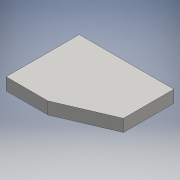
# Autodesk Inventor part: filter top
Saved by Autodesk Inventor 2016 SP1 (Build 200210100, 210)
## iProperties
Created: 2016-05-25
Part Number: filter top
Material: Generic
Document SubType Name: Modeling
Designer: ubik
Density: 1 g/cm^3
Appearance: Default
Author: ubik
Autodesk Inventor part; units mm, degrees
ref_plane "YZ Plane" through (0, 0, 0) normal (1, 0, 0) x (0, 1, 0)
ref_plane "XZ Plane" through (0, 0, 0) normal (0, 1, 0) x (-1, 0, 0)
ref_plane "XY Plane" through (0, 0, 0) normal (0, 0, 1) x (1, 0, 0)
sketch "Sketch1" plane through (0, 0, 0) normal (0, 0, 1) x (1, 0, 0)
  line L0 (-136, 105) -> (136, 105)
  line L1 (136, 105) -> (136, -40)
  line L2 (-16, -105) -> (-136, -105)
  line L3 (-136, -105) -> (-136, 105)
  line L4 (-16, -105) -> (136, -40)
  point P0 (0, 0)
  dimension "d0" = 272
  dimension "d1" = 210
  dimension "d2" = 105
  dimension "d3" = 136
  dimension "d4" = 120
  dimension "d5" = 145
  constraints: 10 end point, 2 parallel, 1 horizontal, 1 perpendicular
  measures "d0" distance of L0.start L0.end
  measures "d1" distance of L2.end L0.start
  measures "d2" distance from line of point (0, 0) L2
  measures "d3" distance from line of point (0, 0) L3
  measures "d4" distance from line of L2.start L3
  measures "d5" distance from line of L1.end L0
extrude "Extrusion1" add sketch "Sketch1" along normal blind 35
equation "\"d2\" = 0.5 * d1"
equation "\"d3\" = 0.5 * d0"
body "Solid1"
